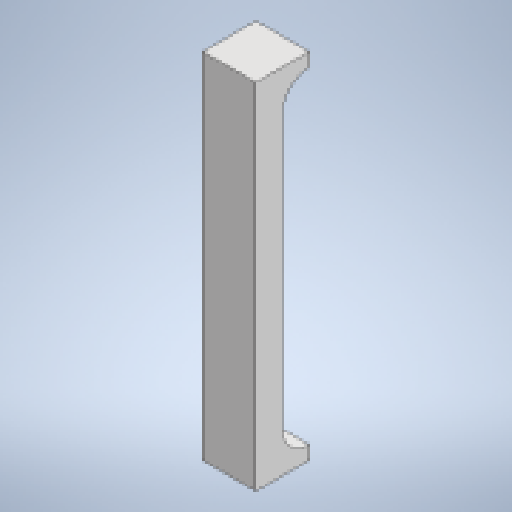
# Autodesk Inventor part: Tope trasero
Saved by Autodesk Inventor 2024 (Build 280153000, 153)
## iProperties
Created: 2025-03-04
Part Number: Tope trasero
Material: Genérico
Document SubType Name: Modeling
Designer: sergi
Density: 1 g/cm^3
Appearance: Valor por defecto
Author: sergi
Autodesk Inventor part; units mm, degrees
ref_plane "YZ Plane" through (0, 0, 0) normal (1, 0, 0) x (0, 1, 0)
sketch "Boceto1" plane through (0, 0, 0) normal (0, 0, 1) x (1, 0, 0)
  line L0 (-5, 0.3078) -> (-5, -2.25) projected
  line L1 (5, -2.25) -> (-5, -2.25) projected
  line L2 (5, 0.3078) -> (5, -2.25) projected
  line L3 (5, 0.3078) -> (-5, 0.3078) projected
  point P0 (0, 0)
extrude "Extrusión1" add sketch "Boceto1" along normal blind 10
sketch "Boceto2" plane through (-5, 0.3078, 0) normal (0, 1, 0) x (1, 0, 0)
  line L0 (10, 0) -> (0, 0) projected
  line L1 (0, 0) -> (0, -10) projected
  line L2 (10, -10) -> (0, -10) projected
  line L3 (10, 0) -> (10, -10) projected
  line L4 (0, 0) -> (0, -10) projected
  line L5 (0, -10) -> (10, -10)
  line L6 (10, -10) -> (10, -5)
  line L7 (10, -5) -> (0, -5)
  line L8 (0, -5) -> (0, -10)
  line L9 (0, -10) -> (10, -10)
  line L10 (10, -10) -> (10, -7)
  line L11 (10, -7) -> (0, -7)
  line L12 (0, -7) -> (0, -10)
  point P0 (5, 0)
  point P1 (0, -5)
  constraints: 16 end point, 4 parallel, 2 horizontal, 2 perpendicular, 1 midpoint
ref_plane "Plano de trabajo1" through (-5, 64.15, -70) normal (0, 1, 0) x (0, 0, 1)
extrude "Extrusión2" add sketch "Boceto2" along normal up to surface (63.8422 mm away) contours L3 L2 L1 L11
sketch "Boceto4" plane through (5, 0.3078, 7) normal (0, 0, -1) x (-1, 0, 0)
  line L0 (10, 63.8422) -> (0, 63.8422) projected
  line L1 (10, 0) -> (10, 63.8422) projected
  line L2 (0, 59.3422) -> (0, 63.8422) projected
  line L3 (10, 63.8422) -> (0, 63.8422) projected
  line L4 (10, 59.3422) -> (10, 63.8422) projected
  line L5 (0, 59.3422) -> (10, 59.3422) projected
  line L6 (10, 61.5922) -> (0, 61.5922) projected
  point P0 (5, -0.3078)
ref_plane "Plano de trabajo2" through (-5, 59.65, 0) normal (0, 0, 1) x (1, 0, 0)
extrude "Extrusión4" add sketch "Boceto4" along normal up to surface (7 mm away) contours L1 L6 L2 L0
